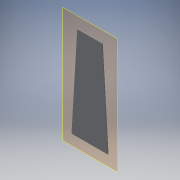
# Autodesk Inventor part: LowerPlate
Saved by Autodesk Inventor 2019.2 (Build 232265000, 265)
## iProperties
Created: 2018-11-25
Part Number: LowerPlate
Material: Generic
Document SubType Name: Modeling
Designer: eroldan
Density: 1 g/cm^3
Appearance: Default
Author: eroldan
Autodesk Inventor part; units mm, degrees
ref_plane "YZ Plane" through (0, 0, 0) normal (1, 0, 0) x (0, 1, 0)
ref_plane "XZ Plane" through (0, 0, 0) normal (0, 1, 0) x (-1, 0, 0)
ref_plane "XY Plane" through (0, 0, 0) normal (0, 0, 1) x (1, 0, 0)
ref_plane "Work Plane1" through (0, 0, 0) normal (0, 0, 1) x (1, 0, 0)
sketch "Sketch1" plane through (0, 0, 0) normal (0, 0, 1) x (1, 0, 0)
  line L0 (143.1602, 7.9375) -> (124.1349, 317.827) construction
  line L1 (145.6, 317.827) -> (20, 317.827) construction
  line L2 (41.4651, 317.827) -> (22.4398, 7.9375) construction
  line L3 (165.6, 7.9375) -> (0, 7.9375) construction
  line L4 (41.4651, 317.827) -> (124.1349, 317.827)
  line L5 (124.1349, 317.827) -> (143.1602, 7.9375)
  line L6 (143.1602, 7.9375) -> (22.4398, 7.9375)
  line L7 (22.4398, 7.9375) -> (41.4651, 317.827)
  line L8 (42.4056, 316.827) -> (123.1944, 316.827)
  line L9 (123.1944, 316.827) -> (142.097, 8.9375)
  line L10 (142.097, 8.9375) -> (23.503, 8.9375)
  line L11 (23.503, 8.9375) -> (42.4056, 316.827)
  point P0 (0, 0)
  dimension "d2" = 1
  constraints: 24 end point, 3 collinear, 2 horizontal, 13 other
  measures "d2" distance between parallel lines of L7 L11
extrude "Extrusion1" add sketch "Sketch1" along normal blind 2 contours L8 L9 L10 L11
chamfer "Chamfer1" distance 1 angle 45 4 edges at (123.1944, 316.827, 1) (42.4056, 316.827, 1) (142.097, 8.9375, 1) (23.503, 8.9375, 1)
sketch "Sketch2" plane through (0, 0, 2) normal (0, 0, 1) x (1, 0, 0)
  line L0 (122.1944, 316.827) -> (43.4056, 316.827) construction
  line L1 (24.503, 8.9375) -> (141.097, 8.9375) construction
  line L2 (43.4056, 316.827) -> (122.1944, 316.827) construction
  line L3 (82.8, 316.827) -> (82.8, 8.9375) construction
  line L4 (141.097, 8.9375) -> (24.503, 8.9375) construction
  point P0 (0, 0)
  point P1 (53.9987, 310.827)
  point P2 (31.008, 14.9375)
  point P3 (111.6013, 310.827)
  point P4 (134.592, 14.9375)
  dimension "d6" = 6
  dimension "d7" = 6
  constraints: 2 end point, 2 midpoint, 2 symmetric about line
  measures "d6" distance from line of L0 point (53.999, 310.827)
  measures "d7" distance from line of L1 point (31.008, 14.938)
hole "Hole1" at (53.9987, 310.827, 2) at (31.008, 14.9375, 2) at (111.6013, 310.827, 2) at (134.592, 14.9375, 2) direction (0, 0, -1) diameter 4 end through all
body "Solid1"
